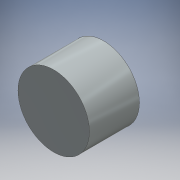
# Autodesk Inventor part: stepperMotor
Saved by Autodesk Inventor 2016 (Build 200138000, 138)
## iProperties
Created: 2015-10-07
Part Number: stepperMotor
Material: Generic
Document SubType Name: Modeling
Designer: alex
Density: 1 g/cm^3
Appearance: Default
Mass: 14.9107 g
Surface Area: 34.8372 cm^2
Volume: 14.9107 cm^3
Author: alex
Autodesk Inventor part; units mm, degrees
ref_plane "YZ Plane" through (0, 0, 0) normal (1, 0, 0) x (0, 1, 0)
ref_plane "XZ Plane" through (0, 0, 0) normal (0, 1, 0) x (-1, 0, 0)
ref_plane "XY Plane" through (0, 0, 0) normal (0, 0, 1) x (1, 0, 0)
sketch "Sketch1" plane through (0, 0, 0) normal (0, 1, 0) x (-1, 0, 0)
  circle A0 centre (0, 0) radius 15
  line L0 (-7.5, 13) -> (-7.4833, 13)
  line L1 (7.4833, 13) -> (7.5, 13)
  point P0 (0, 15)
  dimension "d0" = 30
  constraints: 4 end point, 3 point on circle, 1 centre point, 1 coincident
  measures "d0" diameter of A0
extrude "Extrusion1" add sketch "Sketch1" along normal blind 21
sketch "Sketch2" plane through (0, 21, 0) normal (0, 1, 0) x (1, 0, 0)
  circle A0 centre (-11.25, 0) radius 2.25
  circle A1 centre (0, 0) radius 15 projected
  dimension "d3" = 4.5
  dimension "d4" = 1.5
  constraints: 1 centre point
  measures "d3" diameter of A0
extrude "Extrusion2" add sketch "Sketch2" along normal blind 1 contours A0
sketch "Sketch3" plane through (-11.25, 22, 0) normal (0, 1, 0) x (1, 0, 0)
  circle A0 centre (0, 0) radius 1.5
  point P0 (11.25, 0)
  dimension "d7" = 3
  constraints: 1 centre point
  measures "d7" diameter of A0
extrude "Extrusion3" add sketch "Sketch3" along normal blind 2.5
sketch "Sketch4" plane through (-11.25, 24.5, 0) normal (0, 1, 0) x (1, 0, 0)
  line L0 (1.118, -1) -> (-1.118, -1)
  line L1 (-1.118, 1) -> (1.118, 1)
  line L2 (1.5, -1) -> (-1.882, 1) construction
  line L3 (-1.882, -1) -> (1.0655, 1.0558) construction
  circle A0 centre (0, 0) radius 1.5 projected
  point P0 (11.25, 0)
  point P1 (-0.3302, 0.0823)
  dimension "d10" = 3
  dimension "d11" = 0.5
  dimension "d12" = 0.5
  constraints: 8 end point, 5 point on circle, 2 point on line, 1 horizontal, 1 parallel
  measures "d10" distance of L2.end L1.end
  measures "d11" distance edge to line of A0 L0
  measures "d12" distance edge to line of A0 L1
extrude "Extrusion4" add sketch "Sketch4" along normal blind 6 contours L0 A0 L1
body "Solid1"
